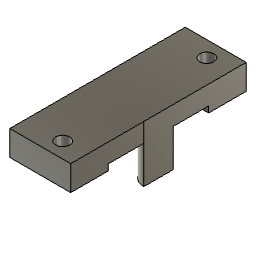
actuator_case_w_table_top_support v2 (Autodesk Fusion 360 archive; units mm, degrees)
design "connection_PS_bottom"
Autodesk Fusion 360 part; units mm, degrees
sketch "Sketch1" plane through (0, 0, 0) normal (0, 0, 1) x (1, 0, 0)
  line L0 (0, 2.9845) -> (0, -2.9845)
  arc A0 (0, 2.9845) -> (0, -2.9845) centre (0, 0) ccw
  dimension "d1" = 5.969
  constraint coincident A0.centre origin
  constraint vertical L0
  measures "d1" diameter of A0
extrude "Extrude1" add sketch "Sketch1" along normal blind 6.35 makes body 1
sketch "Sketch2" plane through (0, 0, 6.35) normal (0, 0, 1) x (-1, 0, 0)
  arc A0 (0, -2.9845) -> (0, 2.9845) centre (0, 0) ccw
  line L0 (0, 2.9845) -> (0, -2.9845)
  line L1 (15.24, -17.78) -> (0, -17.78)
  line L2 (0, -17.78) -> (0, 0)
  line L3 (0, 0) -> (15.24, 0) construction
  circle A1 centre (4.8006, -14.605) radius 1.4224
  circle A2 centre (4.8006, 14.605) radius 1.4224
  line L4 (0, 17.78) -> (0, 0)
  line L5 (15.24, 17.78) -> (0, 17.78)
  line L6 (15.24, -17.78) -> (15.24, 17.78)
  line L7 (0, -6.35) -> (0, 0)
  line L8 (0, -10.16) -> (8.89, -10.16)
  line L9 (11.43, -7.62) -> (11.43, 7.62)
  line L10 (8.89, 10.16) -> (0, 10.16)
  line L11 (2.9845, 0) -> (2.9845, -10.16) construction
  line L12 (2.9845, 0) -> (2.9845, 10.16) construction
  arc A3 (11.43, 7.62) -> (8.89, 10.16) centre (8.89, 7.62) ccw
  arc A4 (8.89, -10.16) -> (11.43, -7.62) centre (8.89, -7.62) ccw
  point P0 (11.43, -10.16)
  dimension "d5" = 17.78
  dimension "d12" = 2.8448
  dimension "d13" = 15.24
  dimension "d14" = 15.24
  dimension "d15" = 3.175
  dimension "d16" = 11.43
  dimension "d18" = 10.16
  dimension "d19" = 10.16
  dimension "d22" = 2.54
  dimension "d35" = 10.4394
  constraint horizontal L1
  constraint vertical L2
  constraint coincident A0.centre L2.end
  constraint symmetric L3 A1 A2
  constraint symmetric A0.centre L3 L2.end
  constraint symmetric L1.start L3 L5.start
  constraint symmetric L1.end L3 L4.start
  constraint midpoint L3.end L6
  constraint coincident L2 L7.start
  constraint coincident L4 A0.centre
  constraint coincident L7 L8.start
  constraint coincident L2 L8.start
  constraint perpendicular L8 L9
  constraint coincident L7 L10.end
  constraint perpendicular L7 L10
  constraint parallel L7 L9
  constraint midpoint A0 L11.start
  constraint coincident L8 L11.end
  constraint tangent A0 L11
  constraint vertical L11
  constraint coincident L10 L12.end
  constraint perpendicular L10 L12
  constraint tangent L9 A3
  constraint tangent L10 A3
  constraint coincident P0 L8
  constraint coincident P0 L9
  constraint tangent L8 A4
  constraint tangent L9 A4
  constraint equal A3 A4
  measures "d5" distance of A0.centre L1.end
  measures "d12" diameter of A1
  measures "d13" distance of L1.start L1.end
  measures "d14" horizontal distance of L4.start L5.start
  measures "d15" distance of L1 A1.centre
  measures "d16" distance of L8.start P0
  measures "d18" distance of L11.start L11.end
  measures "d19" distance of L11.start L12.end
  measures "d22" radius of A3
  measures "d35" distance of A2.centre L6
extrude "Extrude2" add sketch "Sketch2" along normal blind 5.08 separate body contours A0 L2 L4 L7 L8 L9 L10 A3 A4 | L1 L2 L4 L5 L6 L8 L9 L10 A3 A4 makes body 2
extrude "Extrude3" add 1 faces at (-0.8616, -0.4974, 6.35) along direction (0, 0, 1) blind 5.08 on bodies 1 bodies 1 2
extrude "Extrude4" cut sketch "Sketch2" along normal blind 1.2383 contours A0 L2 L4 L7 L8 L9 L10 A3 A4 bodies 1
extrude "Extrude5" cut 1 faces at (-15.24, 5.9267, 8.0433) along direction (1, 0, 0) blind 2.8956 on bodies 1 bodies 1
equation "d5 = ( 1.4 / 2 ) * 1 in"
